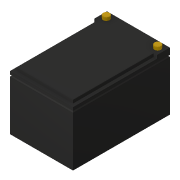
# Autodesk Inventor part: 800-10-ELECTRONICS-BATTERY-12V-12Ah
Saved by Autodesk Inventor 2018.2 (Build 222227000, 227)
## iProperties
Manager: feesmrt
Company: FRANC0R
Created: 2017-12-05
Part Number: 800-10-ELECTRONICS-BATTERY-12V-12Ah
Material: ABS-Kunststoff
Document SubType Name: Modeling
Designer: feesmrt
Density: 1.06 g/cm^3
Appearance: Glatt - schwarz
Project: Rescue Robot
Cost Center: -
Engineer: feesmrt
Authority: feesmrt
Description: Lead-Acid Battery WP12-12 12V 12Ah
Stock Number: 800-10-ELECTRONICS-BATTERY-12V-12Ah
Catalog Web Link: Reichelt
Vendor: https://www.reichelt.de/Blei-Vlies-Akkus-12V-Kung-Long/WP-12-12/3/index.html?ACTION=3&GROUPID=4232&ARTICLE=44421&START=0&OFFSET
Author: feesmrt
Subject: Rescue Robot
Title: Lead-Acid Battery WP12-12 12V 12Ah
Revision Number: 1
Autodesk Inventor part; units mm, degrees
ref_plane "YZ Plane" through (0, 0, 0) normal (1, 0, 0) x (0, 1, 0)
ref_plane "XZ Plane" through (0, 0, 0) normal (0, 1, 0) x (-1, 0, 0)
ref_plane "XY Plane" through (0, 0, 0) normal (0, 0, 1) x (1, 0, 0)
sketch "Skizze1" plane through (0, 0, 0) normal (0, 0, 1) x (1, 0, 0)
  line L0 (-49, -75.5) -> (49, -75.5)
  line L1 (49, -75.5) -> (49, 75.5)
  line L2 (49, 75.5) -> (-49, 75.5)
  line L3 (-49, 75.5) -> (-49, -75.5)
  line L4 (-49, -75.5) -> (49, 75.5) construction
  line L5 (49, -75.5) -> (-49, 75.5) construction
  point P0 (0, 0)
  dimension "d0" = 98
  dimension "d1" = 151
  constraints: 12 end point, 2 midpoint, 2 parallel, 1 horizontal, 1 perpendicular
  measures "d0" distance of L1.end L2.end
  measures "d1" distance of L0.end L1.end
extrude "Grundkörper" add sketch "Skizze1" along normal blind 83
chamfer "Fase" distance 2.5 angle 45 8 edges at (-49, 0, 83) (0, -75.5, 83) (49, 0, 83) (0, 75.5, 83) (0, -75.5, 0) (-49, 0, 0) (49, 0, 0) (0, 75.5, 0)
sketch "Skizze2" plane through (0, 0, 83) normal (0, 0, 1) x (1, 0, 0)
  line L0 (49, -75.5) -> (49, 75.5) projected
  line L1 (49, 75.5) -> (-49, 75.5) projected
  line L2 (-49, -75.5) -> (49, -75.5) projected
  line L3 (-49, 75.5) -> (-49, -75.5) projected
  point P0 (0, 0)
extrude "Cap" add sketch "Skizze2" along normal blind 10
sketch "Skizze3" plane through (0, 0, 93) normal (0, 0, 1) x (1, 0, 0)
  line L0 (44, 55.5) -> (-44, 55.5)
  line L1 (-44, 55.5) -> (-44, -70.5)
  line L2 (-44, -70.5) -> (44, -70.5)
  line L3 (44, -70.5) -> (44, 55.5)
  line L4 (0, 105.7) -> (0, -105.7) construction
  line L5 (49, -75.5) -> (49, 75.5) projected
  line L6 (-49, -75.5) -> (49, -75.5) projected
  line L7 (44, 55.5) -> (49, 55.5)
  line L8 (49, -75.5) -> (49, 75.5) projected
  line L9 (49, 55.5) -> (49, -75.5)
  line L10 (-49, 75.5) -> (-49, -75.5) projected
  line L11 (49, -75.5) -> (-49, -75.5)
  line L12 (-49, -75.5) -> (-49, 55.5)
  line L13 (-44, 55.5) -> (-49, 55.5)
  line L14 (-46.5, -73) -> (-46.5, 73) projected
  line L15 (49, 75.5) -> (-49, 75.5) projected
  point P0 (0, 0)
  dimension "d9" = 5
  dimension "d10" = 5
  dimension "d13" = 20
  constraints: 18 end point, 4 perpendicular, 2 parallel, 2 point on line, 1 collinear, 1 horizontal, 1 other
  measures "d9" distance between parallel lines of L5 L3
  measures "d10" distance between parallel lines of L6 L2
  measures "d13" distance between parallel lines of L15 L0
extrude "Absatz" cut sketch "Skizze3" against normal blind 5 contours L7 L5 L6 L10 L13 L1 L2 L3
sketch "Skizze4" plane through (0, 0, 93) normal (0, 0, 1) x (1, 0, 0)
  line L0 (44, 55.5) -> (49, 55.5) projected
  line L1 (49, 75.5) -> (-49, 75.5) projected
  line L2 (49, 55.5) -> (49, 75.5) projected
  line L3 (-49, 75.5) -> (-49, 55.5) projected
  line L4 (49, 55.5) -> (-49, 55.5)
  line L5 (-49, 75.5) -> (-49, -75.5) projected
  line L6 (-49, 65.5) -> (49, 65.5) construction
  line L7 (49, 75.5) -> (49, -75.5) projected
  line L8 (0, 105.7) -> (0, -105.7) construction
  circle A0 centre (40, 65.5) radius 5
  circle A1 centre (-40, 65.5) radius 5
  point P0 (0, 0)
  dimension "d14" = 10
  dimension "d15" = 80
  constraints: 4 end point, 4 point on line, 2 centre point, 1 equal radius, 1 horizontal, 1 symmetric about line
  measures "d14" diameter of A0
  measures "d15" distance of A1.centre A0.centre
extrude "Connectors" add sketch "Skizze4" along normal blind 5 contours A0 | A1
sketch "Skizze5" plane through (-49, -75.5, 2.5) normal (-1, 0, 0) x (0, 0, 1)
  line L0 (0, 151) -> (78, 151) projected
  line L1 (-2.5, 148.5) -> (-2.5, 2.5) projected
  line L2 (0, 0) -> (78, 0) projected
  line L3 (0, 0) -> (0, 151) projected
  line L4 (0, 0) -> (78, 0) projected
  line L5 (78, 151) -> (78, 0) projected
  line L6 (0, 151) -> (78, 151) projected
  line L7 (78, 151) -> (78, 0) projected
  line L8 (68, 141) -> (68, 95.2469) construction
  line L9 (68, 95.2469) -> (45.5269, 95.2469) construction
  line L10 (45.5269, 95.2469) -> (45.5269, 141) construction
  line L11 (45.5269, 141) -> (68, 141) construction
  line L12 (62.7438, 65.2469) -> (62.7438, 27) construction
  line L13 (62.7438, 27) -> (50.5269, 27) construction
  line L14 (50.5269, 27) -> (50.5269, 65.2469) construction
  line L15 (50.5269, 65.2469) -> (62.7438, 65.2469) construction
  spline S0 degree 2 poles (66.4515, 137.3103) (66.1568, 137.3103) (65.6224, 137.4987) (65.4443, 137.6734) knots 0 0 0 1 2 2 2
  spline S1 degree 2 poles (65.4443, 137.6734) (65.3312, 137.7796) (65.1462, 138.04) (65.0811, 138.1942) knots 0 0 0 1 2 2 2
  spline S2 degree 2 poles (65.0811, 138.1942) (65.016, 138.3518) (64.9406, 138.7183) (64.9406, 138.9444) knots 0 0 0 1 2 2 2
  line L16 (64.9406, 138.9444) -> (64.9406, 139.4994)
  line L17 (64.9406, 139.4994) -> (63.5566, 139.4994)
  line L18 (63.5566, 139.4994) -> (63.5566, 140.5615)
  line L19 (63.5566, 140.5615) -> (67.7842, 140.5615)
  line L20 (67.7842, 140.5615) -> (67.7842, 138.9205)
  spline S3 degree 2 poles (67.7842, 138.9205) (67.7842, 138.5573) (67.6506, 138.0263) (67.5067, 137.8105) knots 0 0 0 1 2 2 2
  spline S4 degree 2 poles (67.5067, 137.8105) (67.3456, 137.5706) (66.8181, 137.3103) (66.4515, 137.3103) knots 0 0 0 1 2 2 2
  spline S5 degree 2 poles (66.4241, 138.3997) (66.6056, 138.3997) (66.8626, 138.571) (66.9106, 138.6875) knots 0 0 0 1 2 2 2
  spline S6 degree 2 poles (66.9106, 138.6875) (66.9756, 138.8382) (66.9962, 139.1123) (66.9962, 139.3487) knots 0 0 0 1 2 2 2
  line L21 (66.9962, 139.3487) -> (66.9962, 139.4994)
  line L22 (66.9962, 139.4994) -> (65.7286, 139.4994)
  line L23 (65.7286, 139.4994) -> (65.7286, 139.4241)
  spline S7 degree 2 poles (65.7286, 139.4241) (65.7286, 139.2768) (65.7355, 139.0095) (65.7526, 138.9102) knots 0 0 0 1 2 2 2
  spline S8 degree 2 poles (65.7526, 138.9102) (65.7663, 138.8245) (65.8485, 138.6361) (65.8999, 138.5847) knots 0 0 0 1 2 2 2
  spline S9 degree 2 poles (65.8999, 138.5847) (66.0027, 138.4751) (66.2322, 138.3997) (66.4241, 138.3997) knots 0 0 0 1 2 2 2
  spline S10 degree 2 poles (65.1496, 133.7405) (64.3617, 133.7405) (63.4572, 134.6004) (63.4572, 135.3849) knots 0 0 0 1 2 2 2
  spline S11 degree 2 poles (63.4572, 135.3849) (63.4572, 136.166) (64.3617, 137.0328) (65.1496, 137.0328) knots 0 0 0 1 2 2 2
  spline S12 degree 2 poles (65.1496, 137.0328) (65.9444, 137.0328) (66.8455, 136.166) (66.8455, 135.3849) knots 0 0 0 1 2 2 2
  spline S13 degree 2 poles (66.8455, 135.3849) (66.8455, 134.6038) (65.941, 133.7405) (65.1496, 133.7405) knots 0 0 0 1 2 2 2
  spline S14 degree 2 poles (65.1428, 134.758) (65.4271, 134.758) (65.8074, 134.8505) (65.9205, 134.9327) knots 0 0 0 1 2 2 2
  spline S15 degree 2 poles (65.9205, 134.9327) (66.0404, 135.0217) (66.1329, 135.2444) (66.1329, 135.3849) knots 0 0 0 1 2 2 2
  spline S16 degree 2 poles (66.1329, 135.3849) (66.1329, 135.5219) (66.0506, 135.7378) (65.9342, 135.8268) knots 0 0 0 1 2 2 2
  spline S17 degree 2 poles (65.9342, 135.8268) (65.8245, 135.9125) (65.4374, 136.0153) (65.1428, 136.0153) knots 0 0 0 1 2 2 2
  spline S18 degree 2 poles (65.1428, 136.0153) (64.8516, 136.0153) (64.4918, 135.9193) (64.3822, 135.8405) knots 0 0 0 1 2 2 2
  spline S19 degree 2 poles (64.3822, 135.8405) (64.2726, 135.7617) (64.1698, 135.5219) (64.1698, 135.378) knots 0 0 0 1 2 2 2
  spline S20 degree 2 poles (64.1698, 135.378) (64.1698, 135.2581) (64.2726, 135.0115) (64.3754, 134.9361) knots 0 0 0 1 2 2 2
  spline S21 degree 2 poles (64.3754, 134.9361) (64.4953, 134.8505) (64.8413, 134.758) (65.1428, 134.758) knots 0 0 0 1 2 2 2
  line L24 (66.7461, 128.4611) -> (63.5566, 129.3929)
  line L25 (63.5566, 129.3929) -> (63.5566, 130.4481)
  line L26 (63.5566, 130.4481) -> (65.619, 131.01)
  line L27 (65.619, 131.01) -> (63.5566, 131.5718)
  line L28 (63.5566, 131.5718) -> (63.5566, 132.627)
  line L29 (63.5566, 132.627) -> (66.7461, 133.552)
  line L30 (66.7461, 133.552) -> (66.7461, 132.5071)
  line L31 (66.7461, 132.5071) -> (64.6357, 132.0172)
  line L32 (64.6357, 132.0172) -> (66.7461, 131.4142)
  line L33 (66.7461, 131.4142) -> (66.7461, 130.5338)
  line L34 (66.7461, 130.5338) -> (64.6357, 129.9651)
  line L35 (64.6357, 129.9651) -> (66.7461, 129.482)
  line L36 (66.7461, 129.482) -> (66.7461, 128.4611)
  spline S22 degree 2 poles (63.4709, 126.4055) (63.4709, 127.31) (64.3343, 128.2727) (65.1325, 128.2727) knots 0 0 0 1 2 2 2
  spline S23 degree 2 poles (65.1325, 128.2727) (65.9136, 128.2727) (66.8455, 127.3751) (66.8455, 126.5665) knots 0 0 0 1 2 2 2
  spline S24 degree 2 poles (66.8455, 126.5665) (66.8455, 125.8368) (66.0541, 125.0968) (65.3209, 125.0968) knots 0 0 0 1 2 2 2
  line L37 (65.3209, 125.0968) -> (64.9612, 125.0968)
  line L38 (64.9612, 125.0968) -> (64.9612, 127.2791)
  spline S25 degree 2 poles (64.9612, 127.2791) (64.7385, 127.2654) (64.4439, 127.1044) (64.3548, 126.9742) knots 0 0 0 1 2 2 2
  spline S26 degree 2 poles (64.3548, 126.9742) (64.2657, 126.8475) (64.1904, 126.5049) (64.1904, 126.3028) knots 0 0 0 1 2 2 2
  spline S27 degree 2 poles (64.1904, 126.3028) (64.1904, 126.1315) (64.2657, 125.7957) (64.3308, 125.6553) knots 0 0 0 1 2 2 2
  spline S28 degree 2 poles (64.3308, 125.6553) (64.3822, 125.5319) (64.509, 125.3264) (64.5569, 125.2613) knots 0 0 0 1 2 2 2
  line L39 (64.5569, 125.2613) -> (64.5569, 125.1551)
  line L40 (64.5569, 125.1551) -> (63.7347, 125.1551)
  spline S29 degree 2 poles (63.7347, 125.1551) (63.6868, 125.2784) (63.6045, 125.4771) (63.5634, 125.6553) knots 0 0 0 1 2 2 2
  spline S30 degree 2 poles (63.5634, 125.6553) (63.5189, 125.8163) (63.4709, 126.1589) (63.4709, 126.4055) knots 0 0 0 1 2 2 2
  spline S31 degree 2 poles (65.5607, 126.0766) (65.8759, 126.0835) (66.2082, 126.361) (66.2082, 126.6453) knots 0 0 0 1 2 2 2
  spline S32 degree 2 poles (66.2082, 126.6453) (66.2082, 126.9365) (65.8588, 127.2654) (65.5607, 127.2826) knots 0 0 0 1 2 2 2
  line L41 (65.5607, 127.2826) -> (65.5607, 126.0766)
  line L42 (65.804, 122.4452) -> (65.804, 122.5274)
  spline S33 degree 2 poles (65.804, 122.5274) (65.8245, 122.5856) (65.8451, 122.8014) (65.8451, 122.9316) knots 0 0 0 1 2 2 2
  spline S34 degree 2 poles (65.8451, 122.9316) (65.8451, 123.0858) (65.7526, 123.4318) (65.6909, 123.5928) knots 0 0 0 1 2 2 2
  line L43 (65.6909, 123.5928) -> (63.5566, 123.5928)
  line L44 (63.5566, 123.5928) -> (63.5566, 124.5864)
  line L45 (63.5566, 124.5864) -> (66.7461, 124.5864)
  line L46 (66.7461, 124.5864) -> (66.7461, 123.5928)
  line L47 (66.7461, 123.5928) -> (66.287, 123.5928)
  spline S35 degree 2 poles (66.287, 123.5928) (66.3487, 123.5243) (66.5406, 123.2845) (66.5988, 123.1852) knots 0 0 0 1 2 2 2
  spline S36 degree 2 poles (66.5988, 123.1852) (66.6639, 123.0755) (66.7564, 122.7877) (66.7564, 122.661) knots 0 0 0 1 2 2 2
  spline S37 degree 2 poles (66.7564, 122.661) (66.7564, 122.613) (66.7495, 122.4931) (66.7461, 122.4452) knots 0 0 0 1 2 2 2
  line L48 (66.7461, 122.4452) -> (65.804, 122.4452)
  line L49 (66.7461, 117.3885) -> (62.3883, 118.9952)
  line L50 (62.3883, 118.9952) -> (62.3883, 120.0641)
  line L51 (62.3883, 120.0641) -> (63.6354, 119.5811)
  line L52 (63.6354, 119.5811) -> (66.7461, 120.7493)
  line L53 (66.7461, 120.7493) -> (66.7461, 119.7078)
  line L54 (66.7461, 119.7078) -> (64.7454, 119.0363)
  line L55 (64.7454, 119.0363) -> (66.7461, 118.4094)
  line L56 (66.7461, 118.4094) -> (66.7461, 117.3885)
  spline S38 degree 2 poles (65.1496, 113.9557) (64.3617, 113.9557) (63.4572, 114.8156) (63.4572, 115.6001) knots 0 0 0 1 2 2 2
  spline S39 degree 2 poles (63.4572, 115.6001) (63.4572, 116.3813) (64.3617, 117.248) (65.1496, 117.248) knots 0 0 0 1 2 2 2
  spline S40 degree 2 poles (65.1496, 117.248) (65.9444, 117.248) (66.8455, 116.3813) (66.8455, 115.6001) knots 0 0 0 1 2 2 2
  spline S41 degree 2 poles (66.8455, 115.6001) (66.8455, 114.819) (65.941, 113.9557) (65.1496, 113.9557) knots 0 0 0 1 2 2 2
  spline S42 degree 2 poles (65.1428, 114.9732) (65.4271, 114.9732) (65.8074, 115.0657) (65.9205, 115.1479) knots 0 0 0 1 2 2 2
  spline S43 degree 2 poles (65.9205, 115.1479) (66.0404, 115.237) (66.1329, 115.4597) (66.1329, 115.6001) knots 0 0 0 1 2 2 2
  spline S44 degree 2 poles (66.1329, 115.6001) (66.1329, 115.7372) (66.0506, 115.953) (65.9342, 116.0421) knots 0 0 0 1 2 2 2
  spline S45 degree 2 poles (65.9342, 116.0421) (65.8245, 116.1277) (65.4374, 116.2305) (65.1428, 116.2305) knots 0 0 0 1 2 2 2
  spline S46 degree 2 poles (65.1428, 116.2305) (64.8516, 116.2305) (64.4918, 116.1346) (64.3822, 116.0558) knots 0 0 0 1 2 2 2
  spline S47 degree 2 poles (64.3822, 116.0558) (64.2726, 115.977) (64.1698, 115.7372) (64.1698, 115.5933) knots 0 0 0 1 2 2 2
  spline S48 degree 2 poles (64.1698, 115.5933) (64.1698, 115.4734) (64.2726, 115.2267) (64.3754, 115.1513) knots 0 0 0 1 2 2 2
  spline S49 degree 2 poles (64.3754, 115.1513) (64.4953, 115.0657) (64.8413, 114.9732) (65.1428, 114.9732) knots 0 0 0 1 2 2 2
  line L57 (63.5566, 110.4681) -> (63.5566, 111.4616)
  line L58 (63.5566, 111.4616) -> (63.9094, 111.4616)
  spline S50 degree 2 poles (63.9094, 111.4616) (63.6936, 111.7186) (63.4675, 112.1502) (63.4675, 112.4483) knots 0 0 0 1 2 2 2
  spline S51 degree 2 poles (63.4675, 112.4483) (63.4675, 112.9211) (64.067, 113.4521) (64.67, 113.4521) knots 0 0 0 1 2 2 2
  line L59 (64.67, 113.4521) -> (66.7461, 113.4521)
  line L60 (66.7461, 113.4521) -> (66.7461, 112.4517)
  line L61 (66.7461, 112.4517) -> (65.1633, 112.4517)
  spline S52 degree 2 poles (65.1633, 112.4517) (64.9167, 112.4517) (64.6015, 112.4277) (64.4953, 112.3798) knots 0 0 0 1 2 2 2
  spline S53 degree 2 poles (64.4953, 112.3798) (64.3959, 112.3318) (64.2931, 112.1434) (64.2931, 111.9721) knots 0 0 0 1 2 2 2
  spline S54 degree 2 poles (64.2931, 111.9721) (64.2931, 111.8693) (64.3959, 111.5815) (64.485, 111.4616) knots 0 0 0 1 2 2 2
  line L62 (64.485, 111.4616) -> (66.7461, 111.4616)
  line L63 (66.7461, 111.4616) -> (66.7461, 110.4681)
  line L64 (66.7461, 110.4681) -> (63.5566, 110.4681)
  line L65 (65.804, 107.5663) -> (65.804, 107.6486)
  spline S55 degree 2 poles (65.804, 107.6486) (65.8245, 107.7068) (65.8451, 107.9226) (65.8451, 108.0528) knots 0 0 0 1 2 2 2
  spline S56 degree 2 poles (65.8451, 108.0528) (65.8451, 108.207) (65.7526, 108.553) (65.6909, 108.714) knots 0 0 0 1 2 2 2
  line L66 (65.6909, 108.714) -> (63.5566, 108.714)
  line L67 (63.5566, 108.714) -> (63.5566, 109.7075)
  line L68 (63.5566, 109.7075) -> (66.7461, 109.7075)
  line L69 (66.7461, 109.7075) -> (66.7461, 108.714)
  line L70 (66.7461, 108.714) -> (66.287, 108.714)
  spline S57 degree 2 poles (66.287, 108.714) (66.3487, 108.6455) (66.5406, 108.4057) (66.5988, 108.3063) knots 0 0 0 1 2 2 2
  spline S58 degree 2 poles (66.5988, 108.3063) (66.6639, 108.1967) (66.7564, 107.9089) (66.7564, 107.7822) knots 0 0 0 1 2 2 2
  spline S59 degree 2 poles (66.7564, 107.7822) (66.7564, 107.7342) (66.7495, 107.6143) (66.7461, 107.5663) knots 0 0 0 1 2 2 2
  line L71 (66.7461, 107.5663) -> (65.804, 107.5663)
  line L72 (63.5566, 104.4898) -> (63.5566, 105.4834)
  line L73 (63.5566, 105.4834) -> (67.9726, 105.4834)
  line L74 (67.9726, 105.4834) -> (67.9726, 104.4898)
  line L75 (67.9726, 104.4898) -> (63.5566, 104.4898)
  line L76 (63.5566, 102.7358) -> (63.5566, 103.7293)
  line L77 (63.5566, 103.7293) -> (66.7461, 103.7293)
  line L78 (66.7461, 103.7293) -> (66.7461, 102.7358)
  line L79 (66.7461, 102.7358) -> (63.5566, 102.7358)
  line L80 (67.2018, 102.7049) -> (67.2018, 103.7567)
  line L81 (67.2018, 103.7567) -> (67.976, 103.7567)
  line L82 (67.976, 103.7567) -> (67.976, 102.7049)
  line L83 (67.976, 102.7049) -> (67.2018, 102.7049)
  line L84 (67.2223, 99.9368) -> (67.2223, 100.0121)
  spline S60 degree 2 poles (67.2223, 100.0121) (67.2394, 100.0704) (67.2943, 100.3136) (67.2943, 100.4198) knots 0 0 0 1 2 2 2
  spline S61 degree 2 poles (67.2943, 100.4198) (67.2943, 100.7213) (67.075, 100.9406) (66.7701, 100.9406) knots 0 0 0 1 2 2 2
  line L85 (66.7701, 100.9406) -> (66.7461, 100.9406)
  line L86 (66.7461, 100.9406) -> (66.7461, 100.1492)
  line L87 (66.7461, 100.1492) -> (66.0541, 100.1492)
  line L88 (66.0541, 100.1492) -> (66.0541, 100.9063)
  line L89 (66.0541, 100.9063) -> (63.5566, 100.9063)
  line L90 (63.5566, 100.9063) -> (63.5566, 101.8998)
  line L91 (63.5566, 101.8998) -> (66.0541, 101.8998)
  line L92 (66.0541, 101.8998) -> (66.0541, 102.2972)
  line L93 (66.0541, 102.2972) -> (66.7461, 102.2972)
  line L94 (66.7461, 102.2972) -> (66.7461, 101.8998)
  line L95 (66.7461, 101.8998) -> (66.8352, 101.8998)
  spline S62 degree 2 poles (66.8352, 101.8998) (67.4176, 101.8998) (68, 101.2866) (68, 100.6631) knots 0 0 0 1 2 2 2
  spline S63 degree 2 poles (68, 100.6631) (68, 100.4472) (67.9692, 100.0738) (67.9418, 99.9368) knots 0 0 0 1 2 2 2
  line L96 (67.9418, 99.9368) -> (67.2223, 99.9368)
  spline S64 degree 2 poles (63.4709, 98.1176) (63.4709, 99.0221) (64.3343, 99.9847) (65.1325, 99.9847) knots 0 0 0 1 2 2 2
  spline S65 degree 2 poles (65.1325, 99.9847) (65.9136, 99.9847) (66.8455, 99.0871) (66.8455, 98.2786) knots 0 0 0 1 2 2 2
  spline S66 degree 2 poles (66.8455, 98.2786) (66.8455, 97.5489) (66.0541, 96.8089) (65.3209, 96.8089) knots 0 0 0 1 2 2 2
  line L97 (65.3209, 96.8089) -> (64.9612, 96.8089)
  line L98 (64.9612, 96.8089) -> (64.9612, 98.9912)
  spline S67 degree 2 poles (64.9612, 98.9912) (64.7385, 98.9775) (64.4439, 98.8165) (64.3548, 98.6863) knots 0 0 0 1 2 2 2
  spline S68 degree 2 poles (64.3548, 98.6863) (64.2657, 98.5596) (64.1904, 98.217) (64.1904, 98.0148) knots 0 0 0 1 2 2 2
  spline S69 degree 2 poles (64.1904, 98.0148) (64.1904, 97.8435) (64.2657, 97.5078) (64.3308, 97.3673) knots 0 0 0 1 2 2 2
  spline S70 degree 2 poles (64.3308, 97.3673) (64.3822, 97.244) (64.509, 97.0384) (64.5569, 96.9733) knots 0 0 0 1 2 2 2
  line L99 (64.5569, 96.9733) -> (64.5569, 96.8671)
  line L100 (64.5569, 96.8671) -> (63.7347, 96.8671)
  spline S71 degree 2 poles (63.7347, 96.8671) (63.6868, 96.9905) (63.6045, 97.1892) (63.5634, 97.3673) knots 0 0 0 1 2 2 2
  spline S72 degree 2 poles (63.5634, 97.3673) (63.5189, 97.5283) (63.4709, 97.8709) (63.4709, 98.1176) knots 0 0 0 1 2 2 2
  spline S73 degree 2 poles (65.5607, 97.7887) (65.8759, 97.7956) (66.2082, 98.0731) (66.2082, 98.3574) knots 0 0 0 1 2 2 2
  spline S74 degree 2 poles (66.2082, 98.3574) (66.2082, 98.6486) (65.8588, 98.9775) (65.5607, 98.9946) knots 0 0 0 1 2 2 2
  line L101 (65.5607, 98.9946) -> (65.5607, 97.7887)
  line L102 (48.9219, 133.0503) -> (48.9219, 139.93)
  line L103 (48.9219, 139.93) -> (59.2372, 139.93)
  line L104 (59.2372, 139.93) -> (59.2372, 137.3386)
  line L105 (59.2372, 137.3386) -> (50.8863, 137.3386)
  line L106 (50.8863, 137.3386) -> (50.8863, 133.0503)
  line L107 (50.8863, 133.0503) -> (48.9219, 133.0503)
  spline S75 degree 2 poles (54.0795, 122.4257) (51.5717, 122.4257) (48.7045, 125.1007) (48.7045, 127.4245) knots 0 0 0 1 2 2 2
  spline S76 degree 2 poles (48.7045, 127.4245) (48.7045, 129.7568) (51.6052, 132.415) (54.0795, 132.415) knots 0 0 0 1 2 2 2
  spline S77 degree 2 poles (54.0795, 132.415) (56.5622, 132.415) (59.4545, 129.7568) (59.4545, 127.4245) knots 0 0 0 1 2 2 2
  spline S78 degree 2 poles (59.4545, 127.4245) (59.4545, 125.1007) (56.5789, 122.4257) (54.0795, 122.4257) knots 0 0 0 1 2 2 2
  spline S79 degree 2 poles (54.0795, 125.1007) (55.0074, 125.1007) (56.3031, 125.4768) (56.7127, 125.8028) knots 0 0 0 1 2 2 2
  spline S80 degree 2 poles (56.7127, 125.8028) (57.139, 126.1289) (57.5068, 126.9648) (57.5068, 127.4162) knots 0 0 0 1 2 2 2
  spline S81 degree 2 poles (57.5068, 127.4162) (57.5068, 127.8927) (57.1641, 128.6701) (56.7294, 129.0295) knots 0 0 0 1 2 2 2
  spline S82 degree 2 poles (56.7294, 129.0295) (56.3282, 129.3472) (54.999, 129.7401) (54.0795, 129.7401) knots 0 0 0 1 2 2 2
  spline S83 degree 2 poles (54.0795, 129.7401) (53.1266, 129.7401) (51.8727, 129.3639) (51.4464, 129.0379) knots 0 0 0 1 2 2 2
  spline S84 degree 2 poles (51.4464, 129.0379) (51.02, 128.7119) (50.6522, 127.8676) (50.6522, 127.4162) knots 0 0 0 1 2 2 2
  spline S85 degree 2 poles (50.6522, 127.4162) (50.6522, 126.9564) (51.0451, 126.1038) (51.4631, 125.7945) knots 0 0 0 1 2 2 2
  spline S86 degree 2 poles (51.4631, 125.7945) (51.9145, 125.4601) (53.1098, 125.1007) (54.0795, 125.1007) knots 0 0 0 1 2 2 2
  line L108 (48.9219, 112.0518) -> (48.9219, 114.5429)
  line L109 (48.9219, 114.5429) -> (56.1108, 118.5219)
  line L110 (56.1108, 118.5219) -> (48.9219, 118.5219)
  line L111 (48.9219, 118.5219) -> (48.9219, 120.8876)
  line L112 (48.9219, 120.8876) -> (59.2372, 120.8876)
  line L113 (59.2372, 120.8876) -> (59.2372, 117.7111)
  line L114 (59.2372, 117.7111) -> (53.3272, 114.4175)
  line L115 (53.3272, 114.4175) -> (59.2372, 114.4175)
  line L116 (59.2372, 114.4175) -> (59.2372, 112.0518)
  line L117 (59.2372, 112.0518) -> (48.9219, 112.0518)
  spline S87 degree 2 poles (49.507, 101.3436) (49.2311, 102.0207) (48.7045, 104.1858) (48.7045, 105.239) knots 0 0 0 1 2 2 2
  spline S88 degree 2 poles (48.7045, 105.239) (48.7045, 107.6716) (51.5132, 110.5555) (54.0879, 110.5555) knots 0 0 0 1 2 2 2
  spline S89 degree 2 poles (54.0879, 110.5555) (56.5121, 110.5555) (59.4378, 107.6716) (59.4378, 105.1638) knots 0 0 0 1 2 2 2
  spline S90 degree 2 poles (59.4378, 105.1638) (59.4378, 103.8681) (58.9446, 102.2464) (58.5267, 101.3854) knots 0 0 0 1 2 2 2
  line L118 (58.5267, 101.3854) -> (56.1025, 101.3854)
  line L119 (56.1025, 101.3854) -> (56.1025, 101.6195)
  spline S91 degree 2 poles (56.1025, 101.6195) (56.2446, 101.8034) (56.7879, 102.5055) (56.9718, 102.8399) knots 0 0 0 1 2 2 2
  spline S92 degree 2 poles (56.9718, 102.8399) (57.1975, 103.2244) (57.5152, 104.2443) (57.5152, 104.8127) knots 0 0 0 1 2 2 2
  spline S93 degree 2 poles (57.5152, 104.8127) (57.5152, 105.4731) (57.0972, 106.5681) (56.6709, 106.9945) knots 0 0 0 1 2 2 2
  spline S94 degree 2 poles (56.6709, 106.9945) (56.2529, 107.4041) (54.974, 107.8806) (54.1297, 107.8806) knots 0 0 0 1 2 2 2
  spline S95 degree 2 poles (54.1297, 107.8806) (52.3241, 107.8806) (50.6021, 106.0666) (50.6021, 104.5034) knots 0 0 0 1 2 2 2
  spline S96 degree 2 poles (50.6021, 104.5034) (50.6021, 104.3613) (50.6188, 103.9935) (50.6271, 103.8514) knots 0 0 0 1 2 2 2
  line L120 (50.6271, 103.8514) -> (52.6584, 103.8514)
  line L121 (52.6584, 103.8514) -> (52.6584, 105.8493)
  line L122 (52.6584, 105.8493) -> (54.5894, 105.8493)
  line L123 (54.5894, 105.8493) -> (54.5894, 101.3436)
  line L124 (54.5894, 101.3436) -> (49.507, 101.3436)
  line L125 (62.6701, 60.9697) -> (59.1701, 61.849)
  line L126 (59.1701, 61.849) -> (59.1701, 62.3708)
  line L127 (59.1701, 62.3708) -> (62.0744, 63.0828)
  line L128 (62.0744, 63.0828) -> (59.1701, 63.7748)
  line L129 (59.1701, 63.7748) -> (59.1701, 64.291)
  line L130 (59.1701, 64.291) -> (62.6701, 65.1845)
  line L131 (62.6701, 65.1845) -> (62.6701, 64.7051)
  line L132 (62.6701, 64.7051) -> (59.7685, 64.0017)
  line L133 (59.7685, 64.0017) -> (62.6701, 63.304)
  line L134 (62.6701, 63.304) -> (62.6701, 62.8303)
  line L135 (62.6701, 62.8303) -> (59.7345, 62.1269)
  line L136 (59.7345, 62.1269) -> (62.6701, 61.4264)
  line L137 (62.6701, 61.4264) -> (62.6701, 60.9697)
  spline S97 degree 2 poles (61.615, 58.3405) (61.3881, 58.3405) (60.9796, 58.5021) (60.8378, 58.6468) knots 0 0 0 1 2 2 2
  spline S98 degree 2 poles (60.8378, 58.6468) (60.6591, 58.8283) (60.4748, 59.319) (60.4748, 59.6934) knots 0 0 0 1 2 2 2
  line L138 (60.4748, 59.6934) -> (60.4748, 60.0876)
  line L139 (60.4748, 60.0876) -> (59.1701, 60.0876)
  line L140 (59.1701, 60.0876) -> (59.1701, 60.5528)
  line L141 (59.1701, 60.5528) -> (62.6701, 60.5528)
  line L142 (62.6701, 60.5528) -> (62.6701, 59.6735)
  spline S99 degree 2 poles (62.6701, 59.6735) (62.6701, 59.3615) (62.568, 58.9247) (62.4517, 58.7574) knots 0 0 0 1 2 2 2
  spline S100 degree 2 poles (62.4517, 58.7574) (62.3184, 58.5617) (61.9071, 58.3405) (61.615, 58.3405) knots 0 0 0 1 2 2 2
  spline S101 degree 2 poles (61.6008, 58.8255) (61.7823, 58.8255) (62.0489, 58.9503) (62.134, 59.0779) knots 0 0 0 1 2 2 2
  spline S102 degree 2 poles (62.134, 59.0779) (62.2077, 59.1885) (62.2673, 59.4835) (62.2673, 59.7019) knots 0 0 0 1 2 2 2
  line L143 (62.2673, 59.7019) -> (62.2673, 60.0876)
  line L144 (62.2673, 60.0876) -> (60.8718, 60.0876)
  line L145 (60.8718, 60.0876) -> (60.8718, 59.7699)
  spline S103 degree 2 poles (60.8718, 59.7699) (60.8718, 59.4863) (60.9626, 59.1375) (61.0817, 59.024) knots 0 0 0 1 2 2 2
  spline S104 degree 2 poles (61.0817, 59.024) (61.1867, 58.9191) (61.4334, 58.8255) (61.6008, 58.8255) knots 0 0 0 1 2 2 2
  line L146 (59.1701, 56.0147) -> (59.1701, 57.7221)
  line L147 (59.1701, 57.7221) -> (59.5274, 57.7221)
  line L148 (59.5274, 57.7221) -> (59.5274, 57.0868)
  line L149 (59.5274, 57.0868) -> (61.8731, 57.0868)
  line L150 (61.8731, 57.0868) -> (61.8731, 57.7221)
  line L151 (61.8731, 57.7221) -> (62.1936, 57.7221)
  spline S105 degree 2 poles (62.1936, 57.7221) (62.1936, 57.3619) (62.3978, 57.0216) (62.6814, 56.9989) knots 0 0 0 1 2 2 2
  line L152 (62.6814, 56.9989) -> (62.6814, 56.6358)
  line L153 (62.6814, 56.6358) -> (59.5274, 56.6358)
  line L154 (59.5274, 56.6358) -> (59.5274, 56.0147)
  line L155 (59.5274, 56.0147) -> (59.1701, 56.0147)
  line L156 (59.1701, 53.2124) -> (59.1701, 55.3708)
  line L157 (59.1701, 55.3708) -> (59.6664, 55.3708)
  spline S106 degree 2 poles (59.6664, 55.3708) (59.8848, 55.1383) (60.2904, 54.7242) (60.5088, 54.5256) knots 0 0 0 1 2 2 2
  spline S107 degree 2 poles (60.5088, 54.5256) (60.9484, 54.1257) (61.476, 53.8336) (61.7568, 53.8336) knots 0 0 0 1 2 2 2
  spline S108 degree 2 poles (61.7568, 53.8336) (61.9043, 53.8336) (62.1255, 53.9243) (62.1964, 54.0066) knots 0 0 0 1 2 2 2
  spline S109 degree 2 poles (62.1964, 54.0066) (62.2673, 54.0888) (62.3382, 54.3044) (62.3382, 54.4349) knots 0 0 0 1 2 2 2
  spline S110 degree 2 poles (62.3382, 54.4349) (62.3382, 54.5597) (62.2758, 54.8149) (62.2276, 54.9312) knots 0 0 0 1 2 2 2
  spline S111 degree 2 poles (62.2276, 54.9312) (62.1879, 55.0305) (62.0744, 55.2148) (62.0347, 55.2716) knots 0 0 0 1 2 2 2
  line L158 (62.0347, 55.2716) -> (62.0347, 55.2971)
  line L159 (62.0347, 55.2971) -> (62.5339, 55.2971)
  spline S112 degree 2 poles (62.5339, 55.2971) (62.6048, 55.1524) (62.7438, 54.6334) (62.7438, 54.4008) knots 0 0 0 1 2 2 2
  spline S113 degree 2 poles (62.7438, 54.4008) (62.7438, 53.9101) (62.2248, 53.3571) (61.7823, 53.3571) knots 0 0 0 1 2 2 2
  spline S114 degree 2 poles (61.7823, 53.3571) (61.5753, 53.3571) (61.2292, 53.4535) (61.0817, 53.5386) knots 0 0 0 1 2 2 2
  spline S115 degree 2 poles (61.0817, 53.5386) (60.9286, 53.6237) (60.6279, 53.8704) (60.4833, 54.0066) knots 0 0 0 1 2 2 2
  spline S116 degree 2 poles (60.4833, 54.0066) (60.2422, 54.2278) (59.726, 54.7695) (59.5757, 54.9312) knots 0 0 0 1 2 2 2
  line L160 (59.5757, 54.9312) -> (59.5757, 53.2124)
  line L161 (59.5757, 53.2124) -> (59.1701, 53.2124)
  line L162 (60.4889, 51.4624) -> (60.4889, 52.787)
  line L163 (60.4889, 52.787) -> (60.9144, 52.787)
  line L164 (60.9144, 52.787) -> (60.9144, 51.4624)
  line L165 (60.9144, 51.4624) -> (60.4889, 51.4624)
  line L166 (59.1701, 49.0147) -> (59.1701, 50.7221)
  line L167 (59.1701, 50.7221) -> (59.5274, 50.7221)
  line L168 (59.5274, 50.7221) -> (59.5274, 50.0868)
  line L169 (59.5274, 50.0868) -> (61.8731, 50.0868)
  line L170 (61.8731, 50.0868) -> (61.8731, 50.7221)
  line L171 (61.8731, 50.7221) -> (62.1936, 50.7221)
  spline S117 degree 2 poles (62.1936, 50.7221) (62.1936, 50.3619) (62.3978, 50.0216) (62.6814, 49.9989) knots 0 0 0 1 2 2 2
  line L172 (62.6814, 49.9989) -> (62.6814, 49.6358)
  line L173 (62.6814, 49.6358) -> (59.5274, 49.6358)
  line L174 (59.5274, 49.6358) -> (59.5274, 49.0147)
  line L175 (59.5274, 49.0147) -> (59.1701, 49.0147)
  line L176 (59.1701, 46.2124) -> (59.1701, 48.3708)
  line L177 (59.1701, 48.3708) -> (59.6664, 48.3708)
  spline S118 degree 2 poles (59.6664, 48.3708) (59.8848, 48.1383) (60.2904, 47.7242) (60.5088, 47.5256) knots 0 0 0 1 2 2 2
  spline S119 degree 2 poles (60.5088, 47.5256) (60.9484, 47.1257) (61.476, 46.8336) (61.7568, 46.8336) knots 0 0 0 1 2 2 2
  spline S120 degree 2 poles (61.7568, 46.8336) (61.9043, 46.8336) (62.1255, 46.9243) (62.1964, 47.0066) knots 0 0 0 1 2 2 2
  spline S121 degree 2 poles (62.1964, 47.0066) (62.2673, 47.0888) (62.3382, 47.3044) (62.3382, 47.4349) knots 0 0 0 1 2 2 2
  spline S122 degree 2 poles (62.3382, 47.4349) (62.3382, 47.5597) (62.2758, 47.8149) (62.2276, 47.9312) knots 0 0 0 1 2 2 2
  spline S123 degree 2 poles (62.2276, 47.9312) (62.1879, 48.0305) (62.0744, 48.2148) (62.0347, 48.2716) knots 0 0 0 1 2 2 2
  line L178 (62.0347, 48.2716) -> (62.0347, 48.2971)
  line L179 (62.0347, 48.2971) -> (62.5339, 48.2971)
  spline S124 degree 2 poles (62.5339, 48.2971) (62.6048, 48.1524) (62.7438, 47.6334) (62.7438, 47.4008) knots 0 0 0 1 2 2 2
  spline S125 degree 2 poles (62.7438, 47.4008) (62.7438, 46.9101) (62.2248, 46.3571) (61.7823, 46.3571) knots 0 0 0 1 2 2 2
  spline S126 degree 2 poles (61.7823, 46.3571) (61.5753, 46.3571) (61.2292, 46.4535) (61.0817, 46.5386) knots 0 0 0 1 2 2 2
  spline S127 degree 2 poles (61.0817, 46.5386) (60.9286, 46.6237) (60.6279, 46.8704) (60.4833, 47.0066) knots 0 0 0 1 2 2 2
  spline S128 degree 2 poles (60.4833, 47.0066) (60.2422, 47.2278) (59.726, 47.7695) (59.5757, 47.9312) knots 0 0 0 1 2 2 2
  line L180 (59.5757, 47.9312) -> (59.5757, 46.2124)
  line L181 (59.5757, 46.2124) -> (59.1701, 46.2124)
  line L182 (53.4074, 63.009) -> (53.4074, 64.7165)
  line L183 (53.4074, 64.7165) -> (53.7648, 64.7165)
  line L184 (53.7648, 64.7165) -> (53.7648, 64.0811)
  line L185 (53.7648, 64.0811) -> (56.1104, 64.0811)
  line L186 (56.1104, 64.0811) -> (56.1104, 64.7165)
  line L187 (56.1104, 64.7165) -> (56.4309, 64.7165)
  spline S129 degree 2 poles (56.4309, 64.7165) (56.4309, 64.3563) (56.6351, 64.0159) (56.9188, 63.9932) knots 0 0 0 1 2 2 2
  line L188 (56.9188, 63.9932) -> (56.9188, 63.6302)
  line L189 (56.9188, 63.6302) -> (53.7648, 63.6302)
  line L190 (53.7648, 63.6302) -> (53.7648, 63.009)
  line L191 (53.7648, 63.009) -> (53.4074, 63.009)
  line L192 (53.4074, 60.2067) -> (53.4074, 62.3652)
  line L193 (53.4074, 62.3652) -> (53.9038, 62.3652)
  spline S130 degree 2 poles (53.9038, 62.3652) (54.1222, 62.1326) (54.5277, 61.7185) (54.7461, 61.5199) knots 0 0 0 1 2 2 2
  spline S131 degree 2 poles (54.7461, 61.5199) (55.1858, 61.12) (55.7133, 60.8279) (55.9941, 60.8279) knots 0 0 0 1 2 2 2
  spline S132 degree 2 poles (55.9941, 60.8279) (56.1416, 60.8279) (56.3628, 60.9187) (56.4337, 61.0009) knots 0 0 0 1 2 2 2
  spline S133 degree 2 poles (56.4337, 61.0009) (56.5047, 61.0832) (56.5756, 61.2987) (56.5756, 61.4292) knots 0 0 0 1 2 2 2
  spline S134 degree 2 poles (56.5756, 61.4292) (56.5756, 61.554) (56.5132, 61.8093) (56.4649, 61.9255) knots 0 0 0 1 2 2 2
  spline S135 degree 2 poles (56.4649, 61.9255) (56.4252, 62.0248) (56.3118, 62.2092) (56.2721, 62.2659) knots 0 0 0 1 2 2 2
  line L194 (56.2721, 62.2659) -> (56.2721, 62.2914)
  line L195 (56.2721, 62.2914) -> (56.7713, 62.2914)
  spline S136 degree 2 poles (56.7713, 62.2914) (56.8422, 62.1468) (56.9812, 61.6277) (56.9812, 61.3952) knots 0 0 0 1 2 2 2
  spline S137 degree 2 poles (56.9812, 61.3952) (56.9812, 60.9045) (56.4621, 60.3514) (56.0196, 60.3514) knots 0 0 0 1 2 2 2
  spline S138 degree 2 poles (56.0196, 60.3514) (55.8126, 60.3514) (55.4666, 60.4478) (55.3191, 60.5329) knots 0 0 0 1 2 2 2
  spline S139 degree 2 poles (55.3191, 60.5329) (55.1659, 60.618) (54.8653, 60.8648) (54.7206, 61.0009) knots 0 0 0 1 2 2 2
  spline S140 degree 2 poles (54.7206, 61.0009) (54.4795, 61.2221) (53.9633, 61.7639) (53.813, 61.9255) knots 0 0 0 1 2 2 2
  line L196 (53.813, 61.9255) -> (53.813, 60.2067)
  line L197 (53.813, 60.2067) -> (53.4074, 60.2067)
  line L198 (56.9074, 57.101) -> (53.4074, 58.3064)
  line L199 (53.4074, 58.3064) -> (53.4074, 58.8084)
  line L200 (53.4074, 58.8084) -> (56.9074, 60.0139)
  line L201 (56.9074, 60.0139) -> (56.9074, 59.5147)
  line L202 (56.9074, 59.5147) -> (54.0002, 58.5447)
  line L203 (54.0002, 58.5447) -> (56.9074, 57.5746)
  line L204 (56.9074, 57.5746) -> (56.9074, 57.101)
  line L205 (53.4074, 53.3798) -> (53.4074, 55.0872)
  line L206 (53.4074, 55.0872) -> (53.7648, 55.0872)
  line L207 (53.7648, 55.0872) -> (53.7648, 54.4519)
  line L208 (53.7648, 54.4519) -> (56.1104, 54.4519)
  line L209 (56.1104, 54.4519) -> (56.1104, 55.0872)
  line L210 (56.1104, 55.0872) -> (56.4309, 55.0872)
  spline S141 degree 2 poles (56.4309, 55.0872) (56.4309, 54.727) (56.6351, 54.3866) (56.9188, 54.364) knots 0 0 0 1 2 2 2
  line L211 (56.9188, 54.364) -> (56.9188, 54.0009)
  line L212 (56.9188, 54.0009) -> (53.7648, 54.0009)
  line L213 (53.7648, 54.0009) -> (53.7648, 53.3798)
  line L214 (53.7648, 53.3798) -> (53.4074, 53.3798)
  line L215 (53.4074, 50.5775) -> (53.4074, 52.7359)
  line L216 (53.4074, 52.7359) -> (53.9038, 52.7359)
  spline S142 degree 2 poles (53.9038, 52.7359) (54.1222, 52.5033) (54.5277, 52.0892) (54.7461, 51.8907) knots 0 0 0 1 2 2 2
  spline S143 degree 2 poles (54.7461, 51.8907) (55.1858, 51.4908) (55.7133, 51.1986) (55.9941, 51.1986) knots 0 0 0 1 2 2 2
  spline S144 degree 2 poles (55.9941, 51.1986) (56.1416, 51.1986) (56.3628, 51.2894) (56.4337, 51.3717) knots 0 0 0 1 2 2 2
  spline S145 degree 2 poles (56.4337, 51.3717) (56.5047, 51.4539) (56.5756, 51.6695) (56.5756, 51.7999) knots 0 0 0 1 2 2 2
  spline S146 degree 2 poles (56.5756, 51.7999) (56.5756, 51.9247) (56.5132, 52.18) (56.4649, 52.2963) knots 0 0 0 1 2 2 2
  spline S147 degree 2 poles (56.4649, 52.2963) (56.4252, 52.3956) (56.3118, 52.5799) (56.2721, 52.6366) knots 0 0 0 1 2 2 2
  line L217 (56.2721, 52.6366) -> (56.2721, 52.6622)
  line L218 (56.2721, 52.6622) -> (56.7713, 52.6622)
  spline S148 degree 2 poles (56.7713, 52.6622) (56.8422, 52.5175) (56.9812, 51.9985) (56.9812, 51.7659) knots 0 0 0 1 2 2 2
  spline S149 degree 2 poles (56.9812, 51.7659) (56.9812, 51.2752) (56.4621, 50.7221) (56.0196, 50.7221) knots 0 0 0 1 2 2 2
  spline S150 degree 2 poles (56.0196, 50.7221) (55.8126, 50.7221) (55.4666, 50.8186) (55.3191, 50.9037) knots 0 0 0 1 2 2 2
  spline S151 degree 2 poles (55.3191, 50.9037) (55.1659, 50.9887) (54.8653, 51.2355) (54.7206, 51.3717) knots 0 0 0 1 2 2 2
  spline S152 degree 2 poles (54.7206, 51.3717) (54.4795, 51.5929) (53.9633, 52.1346) (53.813, 52.2963) knots 0 0 0 1 2 2 2
  line L219 (53.813, 52.2963) -> (53.813, 50.5775)
  line L220 (53.813, 50.5775) -> (53.4074, 50.5775)
  line L221 (53.4074, 50.3875) -> (56.9074, 49.2076)
  line L222 (56.9074, 49.2076) -> (56.9074, 48.6346)
  line L223 (56.9074, 48.6346) -> (53.4074, 47.4547)
  line L224 (53.4074, 47.4547) -> (53.4074, 47.9454)
  line L225 (53.4074, 47.9454) -> (54.3859, 48.2631)
  line L226 (54.3859, 48.2631) -> (54.3859, 49.599)
  line L227 (54.3859, 49.599) -> (53.4074, 49.9166)
  line L228 (53.4074, 49.9166) -> (53.4074, 50.3875)
  line L229 (54.783, 48.3907) -> (56.4309, 48.9324)
  line L230 (56.4309, 48.9324) -> (54.783, 49.4713)
  line L231 (54.783, 49.4713) -> (54.783, 48.3907)
  line L232 (53.4074, 45.0949) -> (53.4074, 45.5374)
  line L233 (53.4074, 45.5374) -> (54.905, 45.5374)
  spline S153 degree 2 poles (54.905, 45.5374) (55.0865, 45.5374) (55.3985, 45.5714) (55.4921, 45.6225) knots 0 0 0 1 2 2 2
  spline S154 degree 2 poles (55.4921, 45.6225) (55.5914, 45.6764) (55.6878, 45.8692) (55.6878, 46.0337) knots 0 0 0 1 2 2 2
  spline S155 degree 2 poles (55.6878, 46.0337) (55.6878, 46.1982) (55.5119, 46.5471) (55.3701, 46.7144) knots 0 0 0 1 2 2 2
  line L234 (55.3701, 46.7144) -> (53.4074, 46.7144)
  line L235 (53.4074, 46.7144) -> (53.4074, 47.1569)
  line L236 (53.4074, 47.1569) -> (57.0634, 47.1569)
  line L237 (57.0634, 47.1569) -> (57.0634, 46.7144)
  line L238 (57.0634, 46.7144) -> (55.7417, 46.7144)
  spline S156 degree 2 poles (55.7417, 46.7144) (55.9204, 46.5159) (56.1076, 46.133) (56.1076, 45.9174) knots 0 0 0 1 2 2 2
  spline S157 degree 2 poles (56.1076, 45.9174) (56.1076, 45.5317) (55.597, 45.0949) (55.112, 45.0949) knots 0 0 0 1 2 2 2
  line L239 (55.112, 45.0949) -> (53.4074, 45.0949)
  point P0 (-2.5, 75.5)
  dimension "d0" = 98
  dimension "d1" = 151
  dimension "d18" = 10
  dimension "d19" = 10
  dimension "d20" = 30
  dimension "d21" = 5
  constraints: 4 other
  measures "d18" distance between parallel lines of L5 L8
  measures "d19" distance between parallel lines of L0 L11
  measures "d20" distance between parallel lines of L9 L15
  measures "d21" distance between parallel lines of L14 L10
extrude "Schrift" cut sketch "Skizze5" against normal blind 0.5 contours S0 S1 S2 L16 L17 L18 L19 L20 S3 S4 | S10 S11 S12 S13 | L24 L25 L26 L27 L28 L29 L30 L31 L32 L33 L34 L35 L36 | S22 S23 S24 L37 L38 S25 S26 S27 S28 L39 L40 S29 S30 | L42 S33 S34 L43 L44 L45 L46 L47 S35 S36 S37 L48 | L49 L50 L51 L52 L53 L54 L55 L56 | S38 S39 S40 S41 | L57 L58 S50 S51 L59 L60 L61 S52 S53 S54 L62 L63 L64 | L65 S55 S56 L66 L67 L68 L69 L70 S57 S58 S59 L71 | L72 L73 L74 L75 | L76 L77 L78 L79 | L80 L81 L82 L83 | L84 S60 S61 L85 L86 L87 L88 L89 L90 L91 L92 L93 L94 L95 S62 S63 L96 | S64 S65 S66 L97 L98 S67 S68 S69 S70 L99 L100 S71 S72 | L102 L103 L104 L105 L106 L107 | S75 S76 S77 S78 | L108 L109 L110 L111 L112 L113 L114 L115 L116 L117 | S87 S88 S89 S90 L118 L119 S91 S92 S93 S94 S95 S96 L120 L121 L122 L123 L124 | L125 L126 L127 L128 L129 L130 L131 L132 L133 L134 L135 L136 L137 | S97 S98 L138 L139 L140 L141 L142 S99 S100 | L146 L147 L148 L149 L150 L151 S105 L152 L153 L154 L155 | L156 L157 S106 S107 S108 S109 S110 S111 L158 L159 S112 S113 S114 S115 S116 L160 L161 | L162 L163 L164 L165 | L166 L167 L168 L169 L170 L171 S117 L172 L173 L174 L175 | L176 L177 S118 S119 S120 S121 S122 S123 L178 L179 S124 S125 S126 S127 S128 L180 L181 | L182 L183 L184 L185 L186 L187 S129 L188 L189 L190 L191 | L192 L193 S130 S131 S132 S133 S134 S135 L194 L195 S136 S137 S138 S139 S140 L196 L197 | L198 L199 L200 L201 L202 L203 L204 | L205 L206 L207 L208 L209 L210 S141 L211 L212 L213 L214 | L215 L216 S142 S143 S144 S145 S146 S147 L217 L218 S148 S149 S150 S151 S152 L219 L220 | L221 L222 L223 L224 L225 L226 L227 L228 | L232 L233 S153 S154 S155 L234 L235 L236 L237 L238 S156 S157 L239
